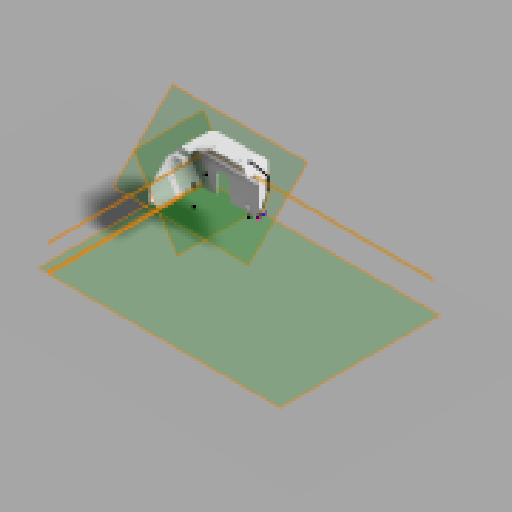
# Autodesk Inventor part: Крыло_универсальное
Saved by Autodesk Inventor 2025 (Build 290162000, 162)
## iProperties
Created: 2025-04-23
Part Number: Крыло_универсальное
Material: Типовые
Document SubType Name: Modeling
Designer: Artem Sannikov
Density: 1 g/cm^3
Appearance: По умолчанию
Author: Artem Sannikov
Autodesk Inventor part; units mm, degrees
ref_plane "YZ Plane" through (0, 0, 0) normal (1, 0, 0) x (0, 1, 0)
ref_plane "XZ Plane" through (0, 0, 0) normal (0, 1, 0) x (-1, 0, 0)
ref_plane "XY Plane" through (0, 0, 0) normal (0, 0, 1) x (1, 0, 0)
sketch "Эскиз1" plane through (0, 0, 0) normal (0, 0, 1) x (1, 0, 0)
  line L0 (-1.5, 74) -> (-1.5, 31) construction
  line L1 (-1.5, 74) -> (-1.5, 94) construction
  line L2 (-1.5, 94) -> (-4.5, 94)
  line L3 (-1.5, 31) -> (-31.5, 31) construction
  line L4 (-1.5, 94) -> (-1.5, 64) construction
  line L5 (-1.5, 64) -> (-31.5, 64) construction
  line L6 (-31.5, 31) -> (-31.5, 64) construction
  line L7 (-31.5, 64) -> (-1.5, 94)
  line L8 (-1.5, 94) -> (1.5, 94)
  line L9 (-28.5, 62.7574) -> (-28.5, 34)
  line L10 (-28.5, 34) -> (-4.5, 34) construction
  line L11 (-4.5, 34) -> (-4.5, 74) construction
  line L12 (-4.5, 74) -> (-4.5, 86.7574) construction
  line L13 (-4.5, 86.7574) -> (-28.5, 62.7574)
  line L14 (-4.5, 34) -> (-1.5, 34) construction
  line L15 (-28.5, 34) -> (-31.5, 34)
  line L16 (-31.5, 34) -> (-31.5, 64)
  line L17 (-1.5, 64) -> (-1.5, 34) construction
  line L18 (-4.5, 86.7574) -> (-1.5, 89.7574)
  line L19 (-1.5, 89.7574) -> (1.5, 89.7574)
  line L20 (1.5, 89.7574) -> (1.5, 94)
  point P0 (0, 0)
  dimension "d0" = 43
  dimension "d1" = 20
  dimension "d2" = 3
  dimension "d3" = 30
  dimension "d4" = 30
  dimension "d5" = 30
  dimension "d6" = 3
  dimension "d7" = 3
  dimension "d8" = 3
  constraints: 42 end point, 6 perpendicular, 4 point on line, 2 horizontal, 2 vertical, 1 collinear, 5 other
  measures "d0" distance of L0.start L0.end
  measures "d1" distance of L0.start L1.end
  measures "d2" distance of L1.end L2.end
  measures "d3" distance of L0.end L3.end
  measures "d4" distance of L1.end L4.end
  measures "d5" distance of L4.end L5.end
  measures "d6" distance of L1.end L8.end
  measures "d7" distance between parallel lines of L6 L9
  measures "d8" distance of L18.end L19.end
sketch "Эскиз2" plane through (0, 0, 0) normal (0, 1, 0) x (-1, 0, 0)
  line L0 (1.5, -20) -> (1.5, 0)
  line L1 (1.5, 0) -> (1.5, 30)
  line L2 (1.5, -20) -> (1.5, -36)
  line L3 (1.5, -36) -> (-9.8137, -47.3137)
  line L4 (-9.8137, -47.3137) -> (-89.8137, -47.3137)
  line L5 (-89.8137, -47.3137) -> (-114.1274, -23)
  line L6 (1.5, -20) -> (-200.5251, -20) construction
  point P0 (0, 0)
  dimension "d9" = 30
  dimension "d10" = 16
  dimension "d11" = 16
  dimension "d12" = 45
  dimension "d13" = 80
  dimension "d14" = 135
  dimension "d18" = 3
  constraints: 14 end point, 2 horizontal, 2 vertical, 1 point on line, 1 other
  measures "d9" distance of L0.end L1.end
  measures "d10" distance of L0.start L2.end
  measures "d11" distance of L2.end L3.end
  measures "d12" angle of L2 L3
  measures "d13" distance of L3.end L4.end
  measures "d14" angle of L5 L4
  measures "d18" distance from line of L6 L5.end
sweep "Сдвиг1" add profiles "Эскиз1" path "Эскиз2" path curves L5 L4 L3 L2 L0 L1
sketch "Эскиз4" plane through (135.3406, 34, -44.2132) normal (0.7071068, 0, 0.7071068) x (0.7071068, 0, -0.7071068)
  line L0 (-30, 55.7574) -> (-33, 55.7574) projected
  line L1 (-3, 28.7574) -> (-30, 55.7574) projected
  line L2 (-3, 0) -> (-3, 28.7574) projected
  line L3 (0, 0) -> (-3, 0) projected
  line L4 (0, 30) -> (0, 0) projected
  line L5 (-30, 60) -> (0, 30) projected
  line L6 (-33, 60) -> (-30, 60) projected
  line L7 (-33, 55.7574) -> (-33, 60) projected
  point P0 (-126.9637, -34)
ref_plane "РабПлоскость1" through (528.5, 69, -20) normal (0, 0, -1) x (-1, 0, 0)
sketch "Эскиз5" plane through (528.5, 69, -20) normal (0, 0, -1) x (-1, 0, 0)
  line L0 (414.3726, 20.7574) -> (416.4939, 20.7574) projected
  line L1 (395.2807, -6.2426) -> (414.3726, 20.7574) projected
  line L2 (395.2807, -35) -> (395.2807, -6.2426) projected
  line L3 (393.1594, -35) -> (395.2807, -35) projected
  line L4 (393.1594, -5) -> (393.1594, -35) projected
  line L5 (414.3726, 25) -> (393.1594, -5) projected
  line L6 (416.4939, 25) -> (414.3726, 25) projected
  line L7 (416.4939, 20.7574) -> (416.4939, 25) projected
  point P0 (528.5, -69)
extrude "Выдавливание1" add sketch "Эскиз5" along normal up to surface surface through (123.6734, 64, -32.5459) normal (-0.7071068, 0, -0.7071068)
sketch "Эскиз6" plane through (-31.5, 34, -48.4264) normal (-1, 0, 0) x (0, 0, 1)
  point P0 (48.4264, -34)
sketch "Эскиз7" plane through (-31.5, 34, -48.4264) normal (-1, 0, 0) x (0, 0, 1)
  line L0 (6.4264, -5.2) -> (6.4264, -12.2) projected
  line L1 (6.4264, -8.7) -> (-23.8236, -8.7) construction
  line L2 (-23.8236, -6.6105) -> (-23.8236, -12.3748) construction
  line L3 (-23.8236, -8.7) -> (-0.8236, -8.7) construction
  line L4 (28.4264, 30) -> (28.4264, 0) projected
  line L5 (-30.0736, -38.2287) -> (28.4264, -38.2287)
  line L6 (28.4264, -38.2287) -> (28.4264, 20.8287)
  line L7 (28.4264, 20.8287) -> (-30.0736, 20.8287)
  line L8 (-30.0736, 20.8287) -> (-30.0736, -38.2287)
  line L9 (-30.0736, -38.2287) -> (28.4264, 20.8287) construction
  line L10 (28.4264, -38.2287) -> (-30.0736, 20.8287) construction
  point P0 (48.4264, -34)
  point P1 (28.4264, 0)
  dimension "d21" = 23
  constraints: 16 end point, 3 midpoint, 3 point on line, 2 horizontal, 2 parallel, 1 perpendicular
  measures "d21" distance of L1.end L3.end
extrude "Выдавливание2" cut sketch "Эскиз7" against normal blind 131.75
sketch "Эскиз8" plane through (-31.5, 34, 30) normal (-1, 0, 0) x (0, 0, 1)
  line L0 (-50, 20.8287) -> (-77.1838, 20.8287) projected
  line L1 (-55.3159, 20.8287) -> (-34.4872, 0)
  line L2 (-50, 0) -> (0, 0) projected
  line L3 (-55.3159, 20.8287) -> (-55.3159, 0)
  line L4 (-50, 0) -> (-72.0919, 0) projected
  line L5 (-55.3159, 0) -> (-34.4872, 0)
  point P0 (-30, -34)
  dimension "d24" = 45
  constraints: 6 end point, 3 point on line, 1 collinear, 1 vertical
  measures "d24" angle of L2 L1
extrude "Выдавливание3" cut sketch "Эскиз8" against normal blind 131.75
sketch "Эскиз9" plane through (-31.5, 34, 30) normal (-1, 0, 0) x (0, 0, 1)
  line L0 (-50, 15.5128) -> (-50, 20.8287) projected
  line L1 (-50, 15.5128) -> (-55.3159, 20.8287)
  line L2 (-50, 20.8287) -> (-77.1838, 20.8287) projected
  line L3 (-50, 20.8287) -> (-50, 15.5128)
  point P0 (-30, -34)
  dimension "d27" = 45
  constraints: 4 end point, 1 perpendicular, 1 point on line
  measures "d27" angle of L1 L0
extrude "Выдавливание4" add sketch "Эскиз9" against normal up to surface (3 mm away)
sketch "Эскиз10" plane through (102.2401, 64, -77.3137) normal (0, 0, -1) x (-1, 0, 0)
  line L0 (0, -30) -> (1.9901, -30) projected
  line L1 (1.9901, -30) -> (22.8189, -9.1713)
  line L2 (103.6102, -9.1713) -> (1.9901, -9.1713) projected
  line L3 (1.9901, -9.1713) -> (1.9901, -30)
  point P0 (102.2401, -64)
  dimension "d30" = 45
  constraints: 4 end point, 1 perpendicular, 1 point on line
  measures "d30" angle of L1 L3
extrude "Выдавливание5" add sketch "Эскиз10" against normal up to surface (3 mm away)
sketch "Эскиз11" plane through (-31.5, 34, 30) normal (-1, 0, 0) x (0, 0, 1)
  line L0 (-50, -47) -> (300, -47) construction
  line L1 (0, 0) -> (47, -47)
  line L2 (15, 15) -> (47, -17)
  line L3 (-78.4264, 30) -> (0, 30) projected
  line L4 (0, 30) -> (15, 15)
  line L5 (47, -47) -> (47, -17)
  line L6 (0, 30) -> (0, 0)
  point P0 (-30, -34)
  dimension "d33" = 45
  constraints: 10 end point, 2 point on line, 2 vertical, 1 collinear, 1 parallel
  measures "d33" angle of L0 L1
extrude "Выдавливание6" add sketch "Эскиз11" against normal up to surface (3 mm away)
ref_plane "РабПлоскость2" through (-1.5, -12, -20) normal (-1, 0, 0) x (0, 0, 1)
sketch "Эскиз12" plane through (-1.5, -12, -20) normal (-1, 0, 0) x (0, 0, 1)
  point P0 (20, 12)
ref_plane "РабПлоскость3" through (-1.5, -13, -20) normal (-0.8429222, -0.5380355, 0) x (0, 0, 1)
sketch "Эскиз13" plane through (-1.5, -13, -20) normal (-0.8429222, -0.5380355, 0) x (0, 0, 1)
  line L0 (0, 0) -> (350, 0) construction
  line L1 (15.5128, 55.7584) -> (50, 55.7584) projected
  line L2 (50, 55.7584) -> (14.5128, 55.7584)
  line L3 (14.5128, 55.7584) -> (14.5128, 0)
  line L4 (14.5128, 0) -> (50, 0)
  line L5 (50, 0) -> (50, 55.7584)
  point P0 (20, 10.1509)
  point P1 (14.5128, 54.9181)
  constraints: 8 end point, 2 parallel, 1 horizontal, 1 perpendicular, 1 point on line
extrude "Выдавливание7" add sketch "Эскиз13" against normal blind 3
ref_plane "РабПлоскость4" through (-31.5, 34, 30) normal (-0.7423006, -0.4738089, -0.4738089) x (0, -0.7071068, 0.7071068)
sketch "Эскиз14" plane through (-31.5, 34, 30) normal (-0.7423006, -0.4738089, -0.4738089) x (0, -0.7071068, 0.7071068)
  line L0 (33.234, -44.7716) -> (0, 0) construction
  line L1 (0, 0) -> (33.234, -44.7716)
  line L2 (66.468, 0) -> (66.468, -2.0102) projected
  line L3 (33.234, -44.7716) -> (32.0927, -45.6189) projected
  line L4 (66.468, 0) -> (33.234, -44.7716)
  line L5 (66.468, 0) -> (0, 0)
  point P0 (2.8284, -54.6998)
  constraints: 6 end point, 1 collinear, 1 horizontal
extrude "Выдавливание8" add sketch "Эскиз14" against normal blind 3
sketch "Эскиз17" plane through (-31.5, 54.8287, -48.4264) normal (-1, 0, 0) x (0, 0, 1)
  point P0 (48.4264, -54.8287)
sketch "Эскиз18" plane through (-31.5, 54.8287, -48.4264) normal (-1, 0, 0) x (0, 0, 1)
  line L0 (28.4264, -45.8287) -> (28.4264, -5.8287) construction
  line L1 (42.9392, -20.8287) -> (42.9392, -67.8287) projected
  line L2 (28.4264, -45.8287) -> (28.4264, -67.8287) construction
  line L3 (28.4264, -45.8287) -> (28.4264, -19.8287) construction
  line L4 (42.9392, -19.8287) -> (28.4264, -19.8287) construction
  line L5 (28.4264, -67.8287) -> (42.9392, -67.8287) construction
  line L6 (23.1105, 0) -> (43.9392, -20.8287) projected
  line L7 (28.4264, -19.8287) -> (8.5977, 0)
  line L8 (23.1105, 0) -> (1.2426, 0) projected
  line L9 (28.4264, -19.8287) -> (42.9392, -19.8287)
  point P0 (48.4264, -54.8287)
  dimension "d44" = 45
  constraints: 12 end point, 2 perpendicular, 2 point on line, 1 horizontal, 1 vertical
  measures "d44" angle of L8 L7
extrude "Выдавливание11" add sketch "Эскиз18" against normal blind 3
sketch "Эскиз19" plane through (-28.5, 35, -5.4872) normal (0, 0, -1) x (-1, 0, 0)
  line L0 (-29.5288, -46.3859) -> (0.0793, 0) projected
  line L1 (-27, -48) -> (-29.5288, -46.3859) projected
  line L2 (3, -1) -> (-27, -48) projected
  line L3 (3, -1) -> (1.4333, 0) projected
  line L4 (0.0793, 0) -> (1.4333, 0) projected
  point P0 (-28.5, -35)
extrude "Выдавливание12" add sketch "Эскиз19" along normal up to surface (14.5128 mm away)
ref_plane "РабПлоскость5" through (263.5, -13, 155) normal (0, -1, 0) x (0, 0, -1)
sketch "Эскиз21" plane through (263.5, -13, 155) normal (0, -1, 0) x (0, 0, -1)
  line L0 (125, -265) -> (78, -295) projected
  line L1 (125, -265) -> (78, -265)
  line L2 (78, -295) -> (78, -265)
  point P0 (155, -263.5)
  constraints: 4 end point, 1 horizontal, 1 perpendicular
extrude "Выдавливание14" add sketch "Эскиз21" against normal blind 3
sketch "Эскиз22" plane through (-28.5, 35, -20) normal (0, 0, -1) x (-1, 0, 0)
  line L0 (-27, -48) -> (-47.2025, -48)
  line L1 (-47.2025, -48) -> (-47.2025, -1)
  line L2 (3, -1) -> (0, -1) projected
  line L3 (3, -1) -> (-27, -48)
  line L4 (3, -1) -> (-0.9849, -1)
  line L5 (-0.9849, -1) -> (-47.2025, -1)
  line L6 (3, -18) -> (3, 29) projected
  line L7 (-47.2025, -1) -> (3, -1)
  line L8 (3, -1) -> (3, 21.829)
  line L9 (3, 21.829) -> (-47.2025, 21.829)
  line L10 (-47.2025, 21.829) -> (-47.2025, -1)
  point P0 (-28.5, -35)
  point P1 (0, -1)
  dimension "d55" = 22.829
  constraints: 18 end point, 3 horizontal, 2 parallel, 2 perpendicular, 2 point on line, 1 vertical
  measures "d55" distance between parallel lines of L9 L5
extrude "Выдавливание15" add sketch "Эскиз22" along normal blind 3
sketch "Эскиз23" plane through (-28.5, 35, -23) normal (0, 0, -1) x (-1, 0, 0)
  line L0 (0, 21.829) -> (0, 3) projected
  line L1 (-47.2025, 21.829) -> (0, 21.829)
  line L2 (0, 21.829) -> (0, 18.829)
  line L3 (0, 18.829) -> (-47.2025, 18.829)
  line L4 (-47.2025, 18.829) -> (-47.2025, 21.829)
  line L5 (-47.2025, 21.829) -> (-161.7193, 21.829)
  line L6 (-161.7193, 21.829) -> (-161.7193, 18.829)
  line L7 (-161.7193, 18.829) -> (-47.2025, 18.829)
  line L8 (-47.2025, 18.829) -> (-47.2025, 21.829)
  line L9 (-161.7193, -1) -> (-161.7193, 27.7574) projected
  point P0 (-28.5, -35)
  point P1 (0, 21.829)
  dimension "d56" = 3
  dimension "d57" = 3
  constraints: 16 end point, 4 parallel, 2 horizontal, 2 perpendicular, 2 point on line
  measures "d56" distance between parallel lines of L1 L3
  measures "d57" distance between parallel lines of L5 L7
extrude "Выдавливание16" add sketch "Эскиз23" along normal up to surface (51.3137 mm away)
sketch "Эскиз24" plane through (-28.5, 56.829, -74.3137) normal (0, 1, 0) x (1, 0, 0)
  line L0 (161.7193, -27.9792) -> (133.7401, 0) projected
  line L1 (161.7193, -27.9792) -> (161.7193, 0) projected
  line L2 (133.7401, 0) -> (161.7193, 0) projected
  line L3 (22.8873, 0) -> (0, -22.8873) projected
  line L4 (0, 0) -> (22.8873, 0) projected
  line L5 (0, -22.8873) -> (0, 0) projected
  point P0 (28.5, -74.3137)
extrude "Выдавливание17" cut sketch "Эскиз24" against normal blind 10
sketch "Эскиз25" plane through (-28.5, 35, -23) normal (0, 0, -1) x (-1, 0, 0)
  circle A0 centre (-79, -9.7) radius 8 construction
  arc A1 (-62.0606, -9.7) -> (-95.9394, -9.7) centre (-79, -9.7) ccw
  line L0 (-62.0606, -9.7) -> (-62.0606, -48)
  line L1 (-95.9394, -9.7) -> (-95.9394, -47)
  line L2 (-161.7193, 18.829) -> (-47.2025, 18.829) projected
  line L3 (-47.2025, 21.829) -> (-47.2025, -48) projected
  line L4 (-161.7193, 18.829) -> (-47.2025, 18.829)
  line L5 (-47.2025, 18.829) -> (-47.2025, -48)
  line L6 (-161.7193, -47) -> (-161.7193, 18.829)
  line L7 (-47.2025, -48) -> (-62.0606, -48)
  line L8 (-95.9394, -47) -> (-161.7193, -47)
  point P0 (-28.5, -35)
  constraints: 14 end point, 3 parallel, 2 point on circle, 2 tangent, 2 vertical, 1 centre point, 1 coincident, 1 horizontal, 1 perpendicular
extrude "Выдавливание18" add sketch "Эскиз25" against normal blind 3
sketch "Эскиз26" plane through (133.2193, -12, -23) normal (1, 0, 0) x (0, 0, -1)
  line L0 (-3, 0) -> (-3, 46) projected
  line L1 (-3, 0) -> (-3, 46)
  line L2 (-3, 46) -> (21.2132, 46) projected
  line L3 (21.2132, 46) -> (-3, 0)
  point P0 (-23, 12)
  constraints: 4 end point, 1 collinear
extrude "Выдавливание19" add sketch "Эскиз26" along normal up to surface (2.1213 mm away)
sketch "Эскиз28" plane through (-28.5, 35, -23) normal (0, 0, 1) x (1, 0, 0)
  line L0 (161.7193, 18.829) -> (47.2025, 18.829) projected
  line L1 (161.7193, 21.829) -> (161.7193, 18.829) projected
  line L2 (47.2025, 21.829) -> (161.7193, 21.829) projected
  line L3 (47.2025, 21.829) -> (47.2025, 18.829) projected
  point P0 (28.5, -35)
extrude "Выдавливание21" add sketch "Эскиз28" along normal blind 3
ref_plane "РабПлоскость6" through (102.2401, 34, -77.3137) normal (0.6626922, -0.3488239, -0.6626922) x (0.7071068, 0, 0.7071068)
sketch "Эскиз29" plane through (102.2401, 34, -77.3137) normal (0.6626922, -0.3488239, -0.6626922) x (0.7071068, 0, 0.7071068)
  line L0 (62.4325, 49.6062) -> (63.9325, 49.083) projected
  line L1 (0, -28.1156) -> (0, 0) projected
  line L2 (63.9325, 49.083) -> (0, 0)
  line L3 (46.8112, -28.1156) -> (46.8112, 0) projected
  line L4 (0, 0) -> (46.8112, 0)
  line L5 (46.8112, 0) -> (63.9325, 49.083)
  point P0 (-17.6256, 76.1524)
  constraints: 6 end point, 1 perpendicular
extrude "Выдавливание22" add sketch "Эскиз29" against normal blind 3
sketch "Эскиз30" plane through (9.8137, 94, -47.3137) normal (0, 1, 0) x (1, 0, 0)
  line L0 (-8.3137, -77.3137) -> (-11.3137, -77.3137) projected
  line L1 (-11.3137, -77.3137) -> (8.6863, -77.3137)
  line L2 (104.3137, -27.3137) -> (104.3137, -24.3137) projected
  line L3 (104.3137, -24.3137) -> (104.3137, -44.3137)
  line L4 (8.6863, -77.3137) -> (8.6863, -59.3137)
  line L5 (104.3137, -44.3137) -> (23.6863, -44.3137)
  line L6 (80, 0) -> (0, 0) projected
  line L7 (104.3137, -24.3137) -> (80, 0) projected
  line L8 (0, 0) -> (-11.3137, -11.3137) projected
  line L9 (-11.3137, -11.3137) -> (-11.3137, -77.3137) projected
  line L10 (23.6863, -44.3137) -> (8.6863, -59.3137)
  point P0 (-9.8137, -47.3137)
  point P1 (8.6863, -44.3137)
  point P2 (104.3137, -27.3137)
  dimension "d81" = 20
  dimension "d82" = 20
  dimension "d83" = 15
  dimension "d84" = 15
  constraints: 10 end point, 2 point on line, 2 vertical, 1 collinear, 1 perpendicular
  measures "d81" distance of L0.end L1.end
  measures "d82" distance of L2.end L3.end
  measures "d83" distance of L5.end point (8.686, -44.314)
  measures "d84" distance of L4.end point (8.686, -44.314)
extrude "Выдавливание23" add sketch "Эскиз30" against normal up to surface (4.2426 mm away)
sketch "Эскиз31" plane through (135.3406, 64, -20) normal (0.8164966, 0.5773503, 0) x (0, 0, -1)
  line L0 (0, 0) -> (0, -62.0537) projected
  line L1 (-17, 36.7423) -> (-17, 33.2782) projected
  line L2 (0, 0) -> (-17, 0)
  line L3 (-17, 0) -> (-17, 36.7423)
  line L4 (-17, 36.7423) -> (0, 36.7423)
  line L5 (0, 36.7423) -> (0, 0)
  line L6 (0, 0) -> (-17, 0)
  line L7 (-17, 0) -> (-17, 14.1421)
  line L8 (-17, 14.1421) -> (0, 14.1421)
  line L9 (0, 14.1421) -> (0, 0)
  point P0 (0, 0.2101)
  point P1 (-17, 33.2782)
  point P2 (0, 14.1421)
  dimension "d87" = 14.1421
  constraints: 16 end point, 4 parallel, 2 horizontal, 2 perpendicular, 1 point on line
  measures "d87" distance between parallel lines of L8 L2
extrude "Выдавливание24" add sketch "Эскиз31" against normal blind 3 contours L4 L5 L8 L3 L1
sketch "Эскиз32" plane through (-1.5, -13, -23) normal (0, -1, 0) x (1, 0, 0)
  line L0 (0, 3) -> (163.4096, 3)
  line L1 (163.4096, 3) -> (163.4096, 150.0456)
  line L2 (163.4096, 150.0456) -> (0, 150.0456)
  line L3 (0, 150.0456) -> (0, 3)
  point P0 (1.5, 23)
  constraints: 8 end point, 2 parallel, 1 horizontal, 1 perpendicular, 1 other
extrude "Выдавливание25" cut sketch "Эскиз32" against normal blind 9.5
sketch "Эскиз33" plane through (-31.5, 34, 30) normal (0, 0, 1) x (1, 0, 0)
  line L0 (30, -44) -> (30, -41.4242) projected
  line L1 (3, 0.8758) -> (30, -41.4242) projected
  line L2 (3, 0) -> (3, 0.8758) projected
  line L3 (0, 0) -> (3, 0) projected
  line L4 (30, -47) -> (0, 0) projected
  line L5 (30, -47) -> (30, -44) projected
  point P0 (31.5, -34)
extrude "Выдавливание26" add sketch "Эскиз33" along normal up to surface surface through (-1.5, -13, 30) normal (0.3993841, 0.254926, -0.8806277)
ref_plane "РабПлоскость7" through (-1.5, -8.5, 320) normal (-1, 0, 0) x (0, 1, 0)
sketch "Эскиз35" plane through (-1.5, -8.5, 320) normal (-1, 0, 0) x (0, 1, 0)
  line L0 (-2.5, 340) -> (-2.5, -10) construction
  line L1 (17.5, -10) -> (17.5, 340) construction
  line L2 (7.5, 340) -> (7.5, -10) construction
  line L3 (7.5, 340) -> (7.5, 300) construction
  circle A0 centre (7.5, 300) radius 6.5
  point P0 (8.5, 320)
  dimension "d94" = 10
  dimension "d95" = 40
  dimension "d96" = 13
  constraints: 4 end point, 1 centre point, 1 coincident, 1 parallel, 1 point on line
  measures "d94" distance between parallel lines of L0 L2
  measures "d95" distance of L2.start L3.end
  measures "d96" diameter of A0
extrude "Выдавливание27" add sketch "Эскиз35" along normal blind 11.601
sketch "Эскиз36" plane through (-1.5, -1, 20) normal (1, 0, 0) x (0, 0, 1)
  arc A0 (-0.99, 6.4242) -> (0.99, 6.4242) centre (0, 0) ccw projected
  circle A1 centre (0, 0) radius 3.25
  point P0 (-20, -1)
  dimension "d99" = 6.5
  constraints: 1 centre point, 1 coincident
  measures "d99" diameter of A1
extrude "Выдавливание28" cut sketch "Эскиз36" against normal blind 15.25
sketch "Эскиз37" plane through (-28.5, 35, -23) normal (0, 0, -1) x (-1, 0, 0)
  line L0 (-537, -26) -> (-47, -26) construction
  line L1 (-557, -46) -> (-27, -46) construction
  line L2 (-557, -36) -> (-27, -36) construction
  circle A0 centre (-138.9318, -36) radius 3.25
  point P0 (-28.5, -35)
  dimension "d102" = 10
  dimension "d103" = 6.5
  constraints: 2 end point, 1 centre point, 1 parallel, 1 point on line
  measures "d102" distance between parallel lines of L1 L2
  measures "d103" diameter of A0
extrude "Выдавливание29" cut sketch "Эскиз37" against normal blind 13.25
ref_plane "РабПлоскость8" through (-1.5, 51.5, 320) normal (-1, 0, 0) x (0, 1, 0)
sketch "Эскиз38" plane through (-1.5, 51.5, 320) normal (-1, 0, 0) x (0, 1, 0)
  line L0 (17.5, 340) -> (17.5, -10) construction
  line L1 (7.5, 340) -> (7.5, -10) construction
  circle A0 centre (-51.5, 300) radius 3.25 projected
  line L2 (-51.5, 300) -> (52.8923, 300) construction
  circle A1 centre (7.5, 300) radius 6.5
  circle A2 centre (7.5, 300) radius 3.25
  point P0 (-51.5, 320)
  dimension "d106" = 10
  dimension "d107" = 13
  dimension "d108" = 6.5
  constraints: 4 end point, 2 centre point, 2 point on line, 1 coincident, 1 horizontal, 1 parallel
  measures "d106" distance between parallel lines of L0 L1
  measures "d107" diameter of A1
  measures "d108" diameter of A2
extrude "Выдавливание30" add sketch "Эскиз38" along normal up to surface (30 mm away) contours A1
sketch "Эскиз39" plane through (-1.5, 59, 20) normal (1, 0, 0) x (0, 0, -1)
  circle A0 centre (0, 0) radius 3.25 projected
  point P0 (20, -59)
extrude "Выдавливание31" cut sketch "Эскиз39" against normal blind 53
fillet "Сопряжение2" radius 9.5 1 edges at (-28.5, 52.5, 20)
sketch "Эскиз41" plane through (102.2401, 34, -77.3137) normal (-0.626249, -0.7433763, -0.2349551) x (0.6626922, -0.3488239, -0.6626922)
  point P0 (-107.1289, 32.3934)
sketch "Эскиз42" plane through (133.2193, -12, -20) normal (1, 0, 0) x (0, 0, -1)
  line L0 (24.2132, 46) -> (0, 0) projected
  line L1 (0, 0) -> (20.8781, 0)
  point P0 (-20, 12)
  constraints: 2 end point, 1 horizontal
sketch "Эскиз43" plane through (-28.5, 35, -23) normal (0, 0, -1) x (-1, 0, 0)
  point P0 (-28.5, -35)
sketch "Эскиз44" plane through (133.2193, -12, -20) normal (1, 0, 0) x (0, 0, -1)
  line L0 (3, 2.7353) -> (1.1284, 2.1437) projected
  line L1 (1.1284, 2.1437) -> (0, 0) projected
  line L2 (3, 0) -> (0, 0) projected
  line L3 (3, 2.7353) -> (3, 0) projected
  point P0 (-20, 12)
sketch "Эскиз45" plane through (9.8137, 94, -47.3137) normal (0, 1, 0) x (1, 0, 0)
  line L0 (118.4558, -27.3137) -> (388.9167, -27.3137) construction
  line L1 (2.359, -37.3137) -> (274.3199, -37.3137) construction
  circle A0 centre (89.3137, -37.3137) radius 3.25
  circle A1 centre (25.3137, -37.3137) radius 3.25
  line L2 (104.3137, -44.3137) -> (104.3137, -24.3137) projected
  point P0 (-9.8137, -47.3137)
  dimension "d120" = 10
  dimension "d121" = 6.5
  dimension "d122" = 15
  dimension "d123" = 64
  constraints: 2 centre point, 2 end point, 2 point on line, 1 equal radius, 1 parallel
  measures "d120" distance between parallel lines of L0 L1
  measures "d121" diameter of A0
  measures "d122" distance from line of L2 A0.centre
  measures "d123" distance of A0.centre A1.centre
extrude "Выдавливание33" cut sketch "Эскиз45" against normal blind 10
chamfer "Фаска5" distance 2 angle 45 1 edges at (-5.0106, -7.5, 20)
fillet "Сопряжение3" radius 2 2 edges at (-5.9174, -0.5035, 26.481) (-5.9174, -0.5035, 13.519)
sketch "Эскиз46" plane through (-31.5, 35, -5.4872) normal (0, -1, 0) x (1, 0, 0)
  line L0 (1.5667, -14.5128) -> (1.5667, 0) projected
  line L1 (0, 0) -> (1.5667, 0) projected
  line L2 (0, -14.5128) -> (0, 0) projected
  line L3 (0, -14.5128) -> (1.5667, -14.5128) projected
  point P0 (31.5, 5.4872)
extrude "Выдавливание34" add sketch "Эскиз46" along normal up to surface surface through (-31.5, 34, -5.4872) normal (-0.5380355, 0.8429222, 0)
sketch "Эскиз47" plane through (67.4394, -12, -23) normal (0, -1, 0) x (1, 0, 0)
  line L0 (65.7799, 0) -> (0, 0) projected
  line L1 (65.7799, 0) -> (65.7799, 3) projected
  line L2 (0, 3) -> (65.7799, 3) projected
  line L3 (0, 0) -> (0, 3) projected
  point P0 (-67.4394, 23)
extrude "Выдавливание35" add sketch "Эскиз47" along normal blind 1
sketch "Эскиз48" plane through (-28.5, 53.829, -23) normal (0, -1, 0) x (1, 0, 0)
  line L0 (0, -28.4264) -> (0, -16.8287) projected
  line L1 (0, -16.8287) -> (-3, -16.8287) projected
  line L2 (-3, -25.4264) -> (-3, -16.8287) projected
  line L3 (0, -28.4264) -> (-3, -25.4264) projected
  line L4 (107.9213, -51.3137) -> (22.8873, -51.3137) projected
  line L5 (25.8873, -54.3137) -> (22.8873, -51.3137) projected
  line L6 (107.9213, -54.3137) -> (25.8873, -54.3137) projected
  line L7 (107.9213, -54.3137) -> (107.9213, -51.3137) projected
  line L8 (128.75, -54.3137) -> (107.9213, -54.3137) projected
  line L9 (107.9213, -51.3137) -> (109.1932, -51.3137)
  line L10 (109.1932, -51.3137) -> (109.1932, -54.3137)
  line L11 (109.1932, -54.3137) -> (107.9213, -54.3137)
  line L12 (107.9213, -54.3137) -> (107.9213, -51.3137)
  point P0 (28.5, 23)
  constraints: 8 end point, 2 parallel, 1 horizontal, 1 perpendicular, 1 point on line
extrude "Выдавливание36" add sketch "Эскиз48" against normal blind 1
sketch "Эскиз49" plane through (-28.5, 56.829, -20) normal (0, 1, 0) x (1, 0, 0)
  point P0 (28.5, -20)
sketch "Эскиз50" plane through (-28.5, 53.829, -23) normal (0, -1, 0) x (1, 0, 0)
  line L0 (0, 3) -> (47.2025, 3) projected
  line L1 (129.4975, -51.3137) -> (108.921, -51.3137) projected
  line L2 (161.7193, 0) -> (0, 0) projected
  line L3 (124.8881, -51.3137) -> (32.1473, -51.3137)
  line L4 (32.1473, -51.3137) -> (32.1473, 0)
  line L5 (32.1473, 0) -> (124.8881, 0)
  line L6 (124.8881, 0) -> (124.8881, -51.3137)
  point P0 (161.7193, 3)
  constraints: 8 end point, 2 parallel, 2 point on line, 1 horizontal, 1 perpendicular
extrude "Выдавливание37" cut sketch "Эскиз50" against normal blind 3.25
chamfer "Фаска6" distance 2 angle 45 4 edges at (3.6473, 55.329, -23) (3.6473, 55.329, -74.3137) (96.3881, 55.329, -74.3137) (96.3881, 55.329, -23)
sketch "Эскиз51" plane through (-31.5, 17, 77) normal (0, 0, 1) x (1, 0, 0)
  line L0 (-3.8785, -23.102) -> (7.1374, -23.102)
  line L1 (7.1374, -23.102) -> (7.1374, -32.6523)
  line L2 (7.1374, -32.6523) -> (-3.8785, -32.6523)
  line L3 (-3.8785, -32.6523) -> (-3.8785, -23.102)
  point P0 (31.5, -17)
  constraints: 8 end point, 2 parallel, 1 horizontal, 1 perpendicular
extrude "Выдавливание38" cut sketch "Эскиз51" along normal blind 3.25
equation "\"d84\" = d83"
